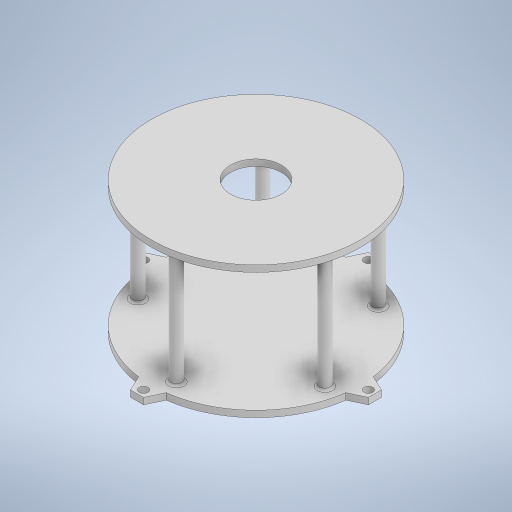
# Autodesk Inventor part: Pieza_base_1
Saved by Autodesk Inventor 2023 (Build 270158000, 158)
## iProperties
Created: 2024-09-21
Part Number: Pieza_base_1
Material: Genérico
Document SubType Name: Sheet Metal
Designer: sebas
Density: 1 g/cm^3
Sheet Metal Rule: Por defecto_mm
Appearance: Valor por defecto
Author: sebas
Autodesk Inventor part; units mm, degrees
ref_plane "YZ Plane" through (0, 0, 0) normal (1, 0, 0) x (0, 1, 0)
ref_plane "XZ Plane" through (0, 0, 0) normal (0, 1, 0) x (-1, 0, 0)
ref_plane "XY Plane" through (0, 0, 0) normal (0, 0, 1) x (1, 0, 0)
sketch "Boceto1" plane through (0, 0, 0) normal (0, 1, 0) x (-1, 0, 0)
  circle A0 centre (0, 0) radius 47.85
  dimension "d0" = 95.7
  constraints: 1 centre point, 1 coincident
  measures "d0" diameter of A0
extrude "Extrusión1" add sketch "Boceto1" along normal blind 2.96
ref_plane "Plano de trabajo1" through (0, 57.66, 0) normal (0, 1, 0) x (1, 0, 0)
sketch "Boceto2" plane through (0, 57.66, 0) normal (0, 1, 0) x (1, 0, 0)
  circle A0 centre (0, 0) radius 47.85 projected
extrude "Extrusión2" add sketch "Boceto2" along normal blind 2.96
sketch "Boceto3" plane through (0, 0, 0) normal (0, -1, 0) x (1, 0, 0)
  circle A0 centre (0, 0) radius 51.5 construction
  circle A1 centre (51.5, 0) radius 2
  line L0 (47.4341, 6.2949) -> (54.5, 3)
  line L1 (54.5, 3) -> (54.5, -3)
  line L2 (54.5, -3) -> (47.4341, -6.2949)
  line L3 (0, 0) -> (0, 96) construction
  line L4 (51.5, 0) -> (55.6486, 0) construction
  arc A2 (47.4341, -6.2949) -> (47.4341, 6.2949) centre (0, 0) ccw
  dimension "d6" = 103
  dimension "d7" = 4
  dimension "d8" = 115
  dimension "d9" = 115
  dimension "d10" = 3
  dimension "d11" = 6
  constraints: 10 end point, 4 point on circle, 3 centre point, 2 coincident, 2 vertical, 1 horizontal, 1 symmetric about line
  measures "d6" diameter of A0
  measures "d7" diameter of A1
  measures "d8" angle of L1 L0
  measures "d9" angle of L2 L1
  measures "d10" distance from line of L1 A1.centre
  measures "d11" distance of L0.end L1.end
extrude "Extrusión3" add sketch "Boceto3" against normal blind 2.96
pattern_circular "Patrón circular1" count 4 over 360 about axis through (0, -10, 0) along (0, 1, 0) of "Extrusión3"
sketch "Boceto4" plane through (0, 0, 0) normal (0, -1, 0) x (1, 0, 0)
  circle A0 centre (0, 0) radius 41 construction
  line L0 (0, 0) -> (20.5, -35.507) construction
  line L1 (0, 0) -> (0, -41) construction
  circle A1 centre (20.5, -35.507) radius 2.5
  dimension "d17" = 82
  dimension "d18" = 30
  dimension "d19" = 5
  constraints: 4 end point, 2 centre point, 2 coincident, 2 point on circle, 1 vertical
  measures "d17" diameter of A0
  measures "d18" angle of L1 L0
  measures "d19" diameter of A1
extrude "Extrusión4" add sketch "Boceto4" against normal up to surface (60.62 mm away)
fillet "Empalme1" radius 1 2 edges at (18, 57.66, -35.507) (18, 2.96, -35.507)
pattern_circular "Patrón circular2" count 5 over 360 about axis through (0, -10, 0) along (0, 1, 0) of "Extrusión4", "Empalme1"
sketch "Boceto5" plane through (0, 60.62, 0) normal (0, 1, 0) x (1, 0, 0)
  circle A0 centre (0, 0) radius 11.6
  dimension "d26" = 23.2
  constraints: 1 centre point, 1 coincident
  measures "d26" diameter of A0
extrude "Extrusión5" cut sketch "Boceto5" against normal up to surface (2.96 mm away)
equation "\"Radio_pliegue\" = Grosor"
equation "\"Anchura_desahogo_plegado\" = Grosor"
equation "\"Profundidad_desahogo_plegado\" = 0.5 * Grosor"
equation "\"Tamaño_destalonado\" = 4 * Grosor"
equation "\"Remanente_mínimo\" = 2 * Grosor"
equation "\"Radiodetransición\" = Radio_pliegue"
equation "\"Tamaño_de_radio_de_Jacobi\" = Radio_pliegue"
equation "\"TamañoSeparación\" = Grosor"
equation "\"Grosor\" = 0.5"
